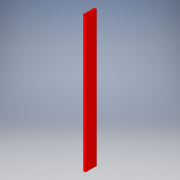
# Autodesk Inventor part: tutup_fin_fix
Saved by Autodesk Inventor 2019 (Build 230136000, 136)
## iProperties
Created: 2020-07-27
Part Number: tutup_fin_fix
Material: Generic
Document SubType Name: Modeling
Designer: Agus Prayudi
Density: 1 g/cm^3
Appearance: Default
Author: Agus Prayudi
Autodesk Inventor part; units mm, degrees
ref_plane "YZ Plane" through (0, 0, 0) normal (1, 0, 0) x (0, 1, 0)
ref_plane "XZ Plane" through (0, 0, 0) normal (0, 1, 0) x (-1, 0, 0)
ref_plane "XY Plane" through (0, 0, 0) normal (0, 0, 1) x (1, 0, 0)
sketch "Sketch2" plane through (0, 0, 0) normal (1, 0, 0) x (0, 1, 0)
  line L0 (-138.9896, 11.158) -> (0, 11.158)
  line L1 (-139.8126, 0.9719) -> (-139.8126, 10.1861)
  line L2 (0, 0) -> (-138.9896, 0)
  line L3 (0, 11.158) -> (0, 0)
  circle A0 centre (-122.5, 5.579) radius 1.5
  circle A1 centre (-70, 5.579) radius 1.5
  circle A2 centre (-17.5, 5.579) radius 1.5
  line L4 (-138.9896, 0) -> (-139.8126, 0)
  line L5 (-139.8126, 0) -> (-139.8126, 0.9719)
  line L6 (-138.9896, 11.158) -> (-139.8126, 11.158)
  line L7 (-139.8126, 11.158) -> (-139.8126, 10.1861)
  constraints: 16 end point, 3 centre point, 3 perpendicular, 1 horizontal, 1 point on line
extrude "Extrusion2" add sketch "Sketch2" along normal blind 2
body "Solid2"
